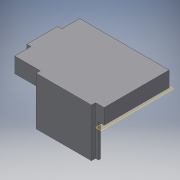
# Autodesk Inventor part: cap
Saved by Autodesk Inventor 2018 (Build 220112000, 112)
## iProperties
Created: 2018-06-27
Part Number: cap
Material: Generic
Document SubType Name: Modeling
Designer: erwin
Density: 1 g/cm^3
Appearance: Default
Author: erwin
Autodesk Inventor part; units mm, degrees
ref_plane "YZ Plane" through (0, 0, 0) normal (1, 0, 0) x (0, 1, 0)
ref_plane "XZ Plane" through (0, 0, 0) normal (0, 1, 0) x (-1, 0, 0)
ref_plane "Work Plane1" through (0, 0, 0) normal (0, 0, 1) x (1, 0, 0)
sketch "Sketch1" plane through (0, 0, 0) normal (0, 0, 1) x (1, 0, 0)
  line L0 (-37.5, -4.8603) -> (-36, -4.8603) construction
  line L1 (-36, -4.8603) -> (-36, -10.5) construction
  line L2 (-36, -10.5) -> (-34, -10.5) construction
  line L3 (-34, -10.5) -> (-34, -13.5) construction
  line L4 (-36, -13.5) -> (-34, -13.5) construction
  line L5 (-36, -10.5) -> (-36, -13.5) construction
  line L6 (-37.5, -15) -> (-37.5, -4.8603) construction
  line L7 (-25.5, -15) -> (-37.5, -15) construction
  line L8 (-25.5, -13.5) -> (-25.5, -15) construction
  line L9 (-34, -13.5) -> (-25.5, -13.5) construction
  line L10 (2.5, -15) -> (-2.5, -15) construction
  line L11 (-2.5, -15) -> (-2.5, -13.5) construction
  line L12 (-2.5, -13.5) -> (-1, -13.5) construction
  line L13 (-1, -13.5) -> (-1, 13.5) construction
  line L14 (1, 13.5) -> (-1, 13.5) construction
  line L15 (1, -13.5) -> (1, 13.5) construction
  line L16 (-1, -13.5) -> (1, -13.5) construction
  line L17 (2.5, 15) -> (2.5, -15) construction
  line L18 (-37.5, 15) -> (2.5, 15) construction
  line L19 (-37.5, 8.1397) -> (-37.5, 15) construction
  line L20 (-36, 8.1397) -> (-37.5, 8.1397) construction
  line L21 (-36, 10.5) -> (-36, 8.1397) construction
  line L22 (-34, 10.5) -> (-36, 10.5) construction
  line L23 (-34, 13.5) -> (-34, 10.5) construction
  line L24 (-34, 13.5) -> (-36, 13.5) construction
  line L25 (-36, 13.5) -> (-36, 10.5) construction
  line L26 (-1, 13.5) -> (-34, 13.5) construction
  line L27 (-36, 13.5) -> (1, 13.5)
  line L28 (1, 13.5) -> (1, -13.5)
  line L29 (-25.5, -15) -> (-2.5, -15)
  line L30 (-2.5, -15) -> (-2.5, -13.5)
  line L31 (-25.5, -13.5) -> (-25.5, -15)
  line L32 (-36, -4.8603) -> (-37.5, -4.8603)
  line L33 (-37.5, -4.8603) -> (-37.5, 8.1397)
  line L34 (-37.5, 8.1397) -> (-36, 8.1397)
  line L35 (-36, -13.5) -> (-36, -4.8603)
  line L36 (-36, 8.1397) -> (-36, 13.5)
  line L37 (1, -13.5) -> (-2.5, -13.5)
  line L38 (-25.5, -13.5) -> (-36, -13.5)
  point P0 (0, 0)
  constraints: 78 end point, 17 horizontal, 13 vertical, 6 parallel, 3 perpendicular, 24 other
extrude "Extrusion1" add sketch "Sketch1" along normal blind 4.25
sketch "Sketch2" plane through (0, 0, 0) normal (0, 0, -1) x (-1, 0, 0)
  line L0 (36, -4.8603) -> (37.5, -4.8603) projected
  line L1 (37.5, -4.8603) -> (37.5, 8.1397) projected
  line L2 (37.5, 8.1397) -> (36, 8.1397) projected
  line L3 (36, 8.1397) -> (36, 13.5) projected
  line L4 (36, 13.5) -> (-1, 13.5) projected
  line L5 (-1, 13.5) -> (-1, -13.5) projected
  line L6 (-1, -13.5) -> (2.5, -13.5) projected
  line L7 (2.5, -13.5) -> (2.5, -15) projected
  line L8 (2.5, -15) -> (25.5, -15) projected
  line L9 (25.5, -15) -> (25.5, -13.5) projected
  line L10 (25.5, -13.5) -> (36, -13.5) projected
  line L11 (36, -13.5) -> (36, -4.8603) projected
  line L12 (25.5, -15) -> (25.5, -13.5) projected
  line L13 (25.5, -15) -> (2.5, -15)
  line L14 (2.5, -15) -> (2.5, -13.5)
  line L15 (4.5, -13.5) -> (23.5, -13.5)
  line L16 (25.5, -13.5) -> (25.5, -15)
  line L17 (36, -13.5) -> (25.5, -13.5) projected
  line L18 (26.5, -13.5) -> (25.5, -13.5)
  line L19 (24.5, -12.5) -> (24.5, -12.5)
  line L20 (24.5, -12.5) -> (26.5, -12.5)
  line L21 (26.5, -12.5) -> (26.5, -13.5)
  line L22 (2.5, -13.5) -> (1.5, -13.5)
  line L23 (1.5, -13.5) -> (1.5, -12.5)
  line L24 (1.5, -12.5) -> (3.5, -12.5)
  line L25 (3.5, -12.5) -> (3.5, -12.5)
  line L26 (24.5, -12.5) -> (23.5, -13.5)
  line L27 (3.5, -12.5) -> (4.5, -13.5)
  point P0 (0, 0)
  point P1 (24.5, -13.5)
  point P2 (3.5, -13.5)
  dimension "d2" = 1
  dimension "d3" = 1
  dimension "d4" = 1
  dimension "d5" = 2
  dimension "d6" = 2
  dimension "d7" = 1
  dimension "d8" = 1
  dimension "d9" = 1
  dimension "d10" = 1
  constraints: 28 end point, 6 parallel, 6 point on line, 3 horizontal, 3 perpendicular, 1 collinear
  measures "d2" distance between parallel lines of L14 L23
  measures "d3" distance between parallel lines of L9 L21
  measures "d4" distance between parallel lines of L15 L20
  measures "d5" distance of L19.end L20.end
  measures "d6" distance of L23.end L24.end
  measures "d7" distance of L19.start point (24.5, -13.5)
  measures "d8" distance of L15.end point (24.5, -13.5)
  measures "d9" distance of L25.end point (3.5, -13.5)
  measures "d10" distance of L15.start point (3.5, -13.5)
ref_plane "Work Plane2" through (-30.5, -15, -15.5) normal (0, 0, -1) x (0, 1, 0)
extrude "Extrusion2" add sketch "Sketch2" along normal up to surface (15.5 mm away) contours L10 L9 L8 L7 L6 L23 L24 L27 L15 L26 L20 L21
sketch "Sketch3" plane through (0, 0, 0) normal (0, 0, -1) x (-1, 0, 0)
  line L0 (1.5, -13.5) -> (1.5, -12.5) projected
  line L1 (1.5, -12.5) -> (3.5, -12.5) projected
  line L2 (3.5, -12.5) -> (4.5, -13.5) projected
  line L3 (4.5, -13.5) -> (23.5, -13.5) projected
  line L4 (23.5, -13.5) -> (24.5, -12.5) projected
  line L5 (24.5, -12.5) -> (26.5, -12.5) projected
  line L6 (26.5, -12.5) -> (26.5, -13.5) projected
  line L7 (26.5, -13.5) -> (36, -13.5) projected
  line L8 (36, -13.5) -> (36, -4.8603) projected
  line L9 (36, -4.8603) -> (37.5, -4.8603) projected
  line L10 (37.5, -4.8603) -> (37.5, 8.1397) projected
  line L11 (37.5, 8.1397) -> (36, 8.1397) projected
  line L12 (36, 8.1397) -> (36, 13.5) projected
  line L13 (36, 13.5) -> (-1, 13.5) projected
  line L14 (-1, 13.5) -> (-1, -13.5) projected
  line L15 (-1, -13.5) -> (1.5, -13.5) projected
  line L16 (36, 8.1397) -> (36, 13.5) projected
  line L17 (36, 13.5) -> (1, 13.5)
  line L18 (1, 13.5) -> (1, -12.5)
  line L19 (1, -12.5) -> (36, -12.5)
  line L20 (37.5, -4.8603) -> (37.5, 8.1397) projected
  line L21 (36, 8.1397) -> (37.5, 8.1397)
  line L22 (37.5, 8.1397) -> (37.5, -4.8603)
  line L23 (37.5, -4.8603) -> (36, -4.8603)
  line L24 (36, -12.5) -> (36, -4.8603)
  line L25 (36, 8.1397) -> (36, 13.5)
  line L26 (5.9109, -12.5) -> (25.9109, -12.5)
  line L27 (25.9109, -12.5) -> (25.9109, -11.5)
  line L28 (25.9109, -11.5) -> (6, -11.5)
  line L29 (36, 12.5) -> (6, 12.5)
  line L30 (1, 12.0898) -> (-8.9254, 12.0898)
  line L31 (6, 12.5) -> (6, -11.5)
  point P0 (0, 0)
  dimension "d13" = 35
  dimension "d14" = 26
  dimension "d16" = 1
  dimension "d17" = 1
  dimension "d18" = 5
  constraints: 28 end point, 5 horizontal, 5 parallel, 3 perpendicular, 3 point on line, 1 vertical
  measures "d13" distance of L19.end L18.end
  measures "d14" distance of L18.end L17.end
  measures "d16" distance between parallel lines of L17 L29
  measures "d17" distance between parallel lines of L26 L28
  measures "d18" distance between parallel lines of L18 L31
extrude "Extrusion3" add sketch "Sketch3" along normal blind 3 contours L15 L14 L30 L18 L19 L0 | L19 L18 L13 L12 L29 L31 L28 L27 L5 L1 | L19 L4 L3 L2 | L14 L13 L18 L30 | L19 L8 L7 L6
move faces "Move1" translate (0, 0, 1) faces at (-22.637, 3.0466, 0)
move faces "Move2" translate (0, 0, 1) faces at (-2.1667, 4.5, -3) (-29.6667, -12.8333, -3)
move faces "Move3" translate (0, 0, 3) faces at (-17.1667, -14.5, -15.5)
move faces "Move4" translate (0, 0, 3) faces at (-20.1667, 2.7132, 4.25)
move faces "Move5" translate (0, 0, 3) faces at (-22.637, 3.0466, 1) (-29.6667, -12.8333, -2) (-2.1667, 4.5, -2)
thicken "Thicken1" operation add thickness 0.2 both sides no extend neighbours yes toward (1, 0, 0) faces at (-25.5, -14, 0.6667) (-29.3333, -13.5, 5.1667) (-36, -10.2868, 6.1667) (-36.5, -4.8603, 5.0833)
thicken "Thicken2" operation add thickness 0.2 both sides no extend neighbours yes toward (0, -1, 0) faces at (-37, 8.1397, 5.0833) (-36, 11.3799, 6.1667) (-11.3333, 13.5, 5.1667) (1, -4.5, 5.1667) (-1, -13.5, 5.1667) (-2.5, -14.5, 0.6667)
move faces "Move6" translate (0, -2, 0) faces at (-36.9333, 7.9397, 5.0833) (-36.3667, -4.6603, 5.0833)
sketch "Sketch4" plane through (-4.5, -13.5, -12.5) normal (0, 0, -1) x (-1, 0, 0)
  line L0 (-3, 1) -> (-3, 0.2) projected
  line L1 (-3, 1) -> (22, 1)
  line L2 (22, 1) -> (22, 0.2)
  line L3 (22, 0.2) -> (-3, 0.2)
  line L4 (-3, 0.2) -> (-3, 1)
  point P0 (-4.5, 13.5)
  constraints: 8 end point, 2 parallel, 1 horizontal, 1 perpendicular
extrude "Extrusion4" cut sketch "Sketch4" against normal blind 3
equation "\"d8\" = d7"
equation "\"d9\" = d7"
equation "\"d10\" = d9"
body "Solid1"
